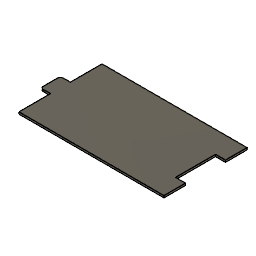
Control board - middle plate v2 (Autodesk Fusion 360 design; units mm, degrees)
Autodesk Fusion 360 part; units mm, degrees
note: some values were not read from the file. Set by a fixed rule: which sketch regions a step uses.
sketch "Sketch1" plane through (0, 0, 0) normal (0, 0, 1) x (1, 0, 0)
  line L0 (-0.9, 44.4476) -> (72, 44.4476)
  line L1 (72, 44.4476) -> (72, 2.6476)
  line L2 (72, 2.6476) -> (-0.9, 2.6476)
  line L3 (-0.9, 2.6476) -> (-0.9, 44.4476)
  line L4 (-0.9, 23.5476) -> (72, 23.5476) construction
  line L5 (72, 13.5476) -> (67, 13.5476)
  line L6 (67, 13.5476) -> (67, 33.5476)
  line L7 (67, 33.5476) -> (72, 33.5476)
  line L8 (72, 33.5476) -> (72, 13.5476)
  line L9 (-0.9, 28.5476) -> (-4.6, 28.5476)
  line L10 (-5.9, 27.2476) -> (-5.9, 19.8476)
  line L11 (-4.6, 18.5476) -> (-0.9, 18.5476)
  line L12 (-0.9, 18.5476) -> (-0.9, 28.5476)
  arc A0 (-4.6, 28.5476) -> (-5.9, 27.2476) centre (-4.6, 27.2476) ccw
  arc A1 (-5.9, 19.8476) -> (-4.6, 18.5476) centre (-4.6, 19.8476) ccw
  point P0 (-5.9, 28.5476)
  point P1 (-5.9, 18.5476)
  dimension "d1" = 72.9
  dimension "d2" = 41.8
  dimension "d5" = 20
  dimension "d6" = 5
  dimension "d7" = 10
  dimension "d8" = 5
  dimension "d9" = 1.3
  constraint horizontal L0
  constraint vertical L1
  constraint horizontal L2
  constraint vertical L3
  constraint midpoint L3 L4.start
  constraint midpoint L1 L4.end
  constraint horizontal L5
  constraint vertical L6
  constraint horizontal L7
  constraint vertical L8
  constraint coincident L1 L5.start
  constraint symmetric L4 L5 L7
  constraint horizontal L9
  constraint vertical L10
  constraint horizontal L11
  constraint vertical L12
  constraint coincident L3 L9.start
  constraint symmetric L4 L9 L11
  constraint coincident P0 L9
  constraint coincident P0 L10
  constraint tangent L9 A0
  constraint tangent L10 A0
  constraint coincident P1 L10
  constraint coincident P1 L11
  constraint tangent L10 A1
  constraint tangent L11 A1
  constraint equal A0 A1
  measures "d1" distance of L0.start L0.end
  measures "d2" distance of L0.end L1.end
  measures "d5" distance of L5.end L6.end
  measures "d6" distance of L6.end L7.end
  measures "d7" distance of P0 P1
  measures "d8" distance of L9.start P0
  measures "d9" radius of A0
extrude "Extrude1" add sketch "Sketch1" along normal blind 1 contours L0 L1 L2 L3 L5 L6 L7 L12 | L3 L9 L10 L11 L12 A0 A1
